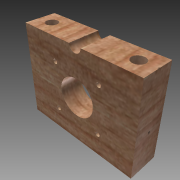
# Autodesk Inventor part: Z_MotorMount_RodHolder_V2
Saved by Autodesk Inventor 2014 (Build 180170000, 170)
## iProperties
Created: 2013-12-13
Part Number: Z_MotorMount_RodHolder_V2
Material: Birch
Document SubType Name: Modeling
Designer: Bram
Density: 0.512 g/cm^3
Appearance: Birch - Natural Medium Gloss
Author: Bram
Autodesk Inventor part; units mm, degrees
ref_plane "YZ Plane" through (0, 0, 0) normal (1, 0, 0) x (0, 1, 0)
ref_plane "XZ Plane" through (0, 0, 0) normal (0, 1, 0) x (-1, 0, 0)
ref_plane "XY Plane" through (0, 0, 0) normal (0, 0, 1) x (1, 0, 0)
sketch "Sketch1" plane through (0, 0, 0) normal (0, 1, 0) x (-1, 0, 0)
  line L0 (-78, 0) -> (-78, -60)
  line L1 (-78, -60) -> (0, -60)
  line L2 (0, -60) -> (0, 0)
  arc A0 (-43, 0) -> (-35, 0) centre (-39, 0) ccw
  circle A1 centre (-39, -30) radius 12
  line L3 (-23.5, -14.5) -> (-54.5, -14.5)
  circle A2 centre (-23.5, -45.5) radius 1.5
  circle A3 centre (-54.5, -45.5) radius 1.5
  circle A4 centre (-54.5, -14.5) radius 1.5
  circle A5 centre (-23.5, -14.5) radius 1.5
  line L4 (0, 0) -> (-35, 0)
  line L5 (-43, 0) -> (-78, 0)
  dimension "d1" = 60
  dimension "d2" = 78
  dimension "d3" = 8
  dimension "d5" = 24
  dimension "d15" = 31
  dimension "d16" = 3
  dimension "d17" = 3
  dimension "d18" = 3
  dimension "d19" = 3
  constraints: 12 end point, 6 centre point, 2 coincident, 2 horizontal, 2 parallel, 2 perpendicular, 2 point on circle
  measures "d1" distance of L0.start L0.end
  measures "d2" distance of L0.end L1.end
  measures "d3" diameter of A0
  measures "d5" diameter of A1
  measures "d15" distance of L3.start L3.end
  measures "d16" diameter of A2
  measures "d17" diameter of A3
  measures "d18" diameter of A4
  measures "d19" diameter of A5
extrude "Extrusion1" add sketch "Sketch1" along normal blind 20
sketch "Sketch2" plane through (78, 0, -60) normal (0, 0, -1) x (-1, 0, 0)
  circle A0 centre (10, 10) radius 4
  circle A1 centre (68, 10) radius 4
  dimension "d24" = 8
  dimension "d25" = 8
  constraints: 2 centre point
  measures "d24" diameter of A0
  measures "d25" diameter of A1
extrude "Extrusion2" cut sketch "Sketch2" against normal blind 100
sketch "Sketch3" plane through (0, 20, 0) normal (0, 1, 0) x (1, 0, 0)
  circle A0 centre (39, 30) radius 12 projected
  circle A1 centre (23.5, 14.5) radius 1.5 projected
  circle A2 centre (54.5, 14.5) radius 1.5 projected
  circle A3 centre (54.5, 45.5) radius 1.5 projected
  circle A4 centre (23.5, 45.5) radius 1.5 projected
  line L0 (60.5, 8.5) -> (17.5, 8.5)
  line L1 (17.5, 8.5) -> (17.5, 51.5)
  line L2 (17.5, 51.5) -> (60.5, 51.5)
  line L3 (60.5, 51.5) -> (60.5, 8.5)
  line L4 (60.5, 8.5) -> (17.5, 51.5) construction
  line L5 (17.5, 8.5) -> (60.5, 51.5) construction
  dimension "d28" = 43
  dimension "d29" = 43
  constraints: 12 end point, 2 midpoint, 2 parallel, 1 horizontal, 1 perpendicular
  measures "d28" distance of L1.end L2.end
  measures "d29" distance of L0.end L1.end
extrude "Extrusion3" cut sketch "Sketch3" against normal blind 5
body "Solid1"
